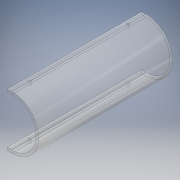
# Autodesk Inventor part: goulotte
Saved by Autodesk Inventor 2017 (Build 210142000, 142)
## iProperties
Created: 2018-04-06
Part Number: goulotte
Material: Generic
Document SubType Name: Modeling
Designer: franc
Density: 1 g/cm^3
Appearance: Default
Author: franc
Autodesk Inventor part; units mm, degrees
ref_plane "YZ Plane" through (0, 0, 0) normal (1, 0, 0) x (0, 1, 0)
ref_plane "XZ Plane" through (0, 0, 0) normal (0, 1, 0) x (-1, 0, 0)
sketch "Sketch1" plane through (0, 0, 0) normal (0, 1, 0) x (-1, 0, 0)
  arc A0 (0, 27) -> (0, -27) centre (0, 0) ccw
  arc A1 (0, 30) -> (0, -30) centre (0, 0) ccw
  line L0 (0, 30) -> (0, 27)
  line L1 (0, -27) -> (0, -30)
  line L2 (0, -30) -> (5, -30)
  line L3 (5, -30) -> (5, -26.533)
  line L4 (5, -26.533) -> (0, -26.533)
  line L5 (0, -26.533) -> (0, -30)
  line L6 (0, 27) -> (5, 27)
  line L7 (5, 27) -> (5, 29.5804)
  line L8 (5, 29.5804) -> (0, 29.5804)
  line L9 (0, 29.5804) -> (0, 27)
  dimension "d0" = 30
  dimension "d1" = 27
  dimension "d31" = 5
  dimension "d32" = 5
  constraints: 20 end point, 6 point on circle, 5 equal length, 2 centre point, 2 coincident, 2 horizontal, 2 perpendicular, 1 vertical
  measures "d0" radius of A1
  measures "d1" radius of A0
  measures "d31" distance of L4.end L3.end
  measures "d32" distance of L8.end L7.end
extrude "Extrusion1" add sketch "Sketch1" along normal blind 150
ref_plane "Work Plane2" through (0, 0, 30) normal (0, 0, 1) x (1, 0, 0)
sketch "Sketch3" plane through (0, 0, 30) normal (0, 0, 1) x (1, 0, 0)
  circle A0 centre (0, 20) radius 1.5
  circle A1 centre (0, 130) radius 1.5
  line L0 (0, 0) -> (30, 0) projected
  line L1 (0, 0) -> (0, 150) projected
  line L2 (30, 150) -> (0, 150) projected
  line L3 (-5, 0) -> (-5, 150) projected
  dimension "d14" = 3
  dimension "d15" = 20
  dimension "d17" = 3
  dimension "d18" = 20
  dimension "d33" = 5
  dimension "d34" = 5
  constraints: 2 centre point
  measures "d14" diameter of A0
  measures "d15" distance from line of L0 A0.centre
  measures "d17" diameter of A1
  measures "d18" distance from line of L2 A1.centre
  measures "d33" distance from line of L3 A1.centre
  measures "d34" distance from line of L3 A0.centre
extrude "Extrusion3" cut sketch "Sketch3" against normal through all
ref_plane "Work Plane3" through (0, 0, -30) normal (0, 0, 1) x (1, 0, 0)
body "Solid1"
